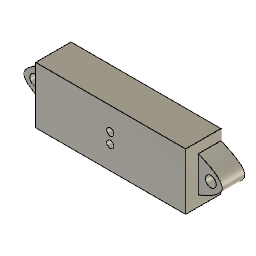
Distance Sensor (Autodesk Fusion 360 design; units mm, degrees)
Autodesk Fusion 360 part; units mm, degrees
note: some values were not read from the file. Set by a fixed rule: which sketch regions a step uses.
sketch "Sketch2" plane through (0, 0, 0) normal (0, 1, 0) x (1, 0, 0)
  line L0 (0, 0) -> (42.015, 0)
  line L1 (42.015, 0) -> (42.015, -15.89)
  line L2 (42.015, -15.89) -> (0, -15.89)
  line L3 (0, -15.89) -> (0, 0)
  circle A0 centre (45.515, -7.945) radius 1.5
  line L4 (42.015, -7.945) -> (48.69, -7.945)
  spline S0 degree 5 poles (42.015, -12.945) (42.5156, -12.7419) (43.4745, -12.3366) (44.7863, -11.7309) (46.2763, -10.9278) (47.6689, -9.93) (48.5399, -8.9364) (48.8392, -7.945) (48.5399, -6.9536) (47.6689, -5.96) (46.2763, -4.9622) (44.7863, -4.1591) (43.4745, -3.5534) (42.5156, -3.1481) (42.015, -2.945) knots 0 0 0 0 0 0 0.1 0.2 0.3 0.4 0.5 0.6 0.7 0.8 0.9 1 1 1 1 1 1
  line L5 (20.92, -15.89) -> (20.92, 0)
  spline S1 degree 5 poles (-0.175, -12.945) (-0.6756, -12.7419) (-1.6345, -12.3366) (-2.9463, -11.7309) (-4.4363, -10.9278) (-5.8289, -9.93) (-6.6999, -8.9364) (-6.9992, -7.945) (-6.6999, -6.9536) (-5.8289, -5.96) (-4.4363, -4.9622) (-2.9463, -4.1591) (-1.6345, -3.5534) (-0.6756, -3.1481) (-0.175, -2.945) knots 0 0 0 0 0 0 0.1 0.2 0.3 0.4 0.5 0.6 0.7 0.8 0.9 1 1 1 1 1 1
  line L6 (40.2192, -13.6735) -> (43.8108, -12.2165)
  line L7 (43.8108, -3.6735) -> (40.2192, -2.2165)
  line L8 (1.6208, -13.6735) -> (-1.9708, -12.2165)
  line L9 (-1.9708, -3.6735) -> (1.6208, -2.2165)
  circle A1 centre (-3.675, -7.945) radius 1.5
  line L10 (-0.175, -7.945) -> (-6.85, -7.945)
  circle A2 centre (20.92, -9.45) radius 1
  circle A3 centre (20.92, -6.45) radius 1
  line L11 (-0.175, -12.945) -> (0, -13.016)
  line L12 (-0.175, -7.945) -> (0, -7.945)
  line L13 (-0.175, -2.945) -> (0, -2.874)
  dimension "d2" = 15.89
  dimension "d3" = 3
  dimension "d5" = 3.5
  dimension "d6" = 10
  dimension "d7" = 2.945
  dimension "d8" = 15.89
  dimension "d19" = 2
  dimension "d20" = 2
  dimension "d21" = 3
  dimension "d22" = 6.45
  dimension "d25" = 49.19
  dimension "d26" = 42.19
  dimension "d27" = 55.54
  dimension "d29" = 7.945
  constraint horizontal L0
  constraint vertical L1
  constraint horizontal L2
  constraint vertical L3
  constraint coincident L0.start L3.end
  constraint midpoint L1 L4.start
  constraint perpendicular L1 L4
  constraint coincident L1 S0.start
  constraint coincident L1 S0.end
  constraint coincident L2 L5.start
  constraint coincident L0 L5.end
  constraint perpendicular L0 L5
  constraint midpoint S0.start L6
  constraint midpoint S0.end L7
  constraint symmetric A0 L5 A1
  constraint symmetric L4.start L5 L10.start
  constraint symmetric L4.end L5 L10.end
  constraint symmetric S0.start L5 S1.start
  constraint symmetric S0.end L5 S1.end
  constraint symmetric L5 L6.start L8.start
  constraint symmetric L5 L6.end L8.end
  constraint symmetric L5 L7.start L9.start
  constraint symmetric L5 L7.end L9.end
  constraint coincident L5 A2.centre
  constraint coincident L5 A3.centre
  constraint coincident L8 L11.end
  constraint coincident L3 L11.end
  constraint midpoint L3 L12.end
  constraint perpendicular L3 L12
  constraint coincident L9 L13.end
  constraint coincident L3 L13.end
  measures "d2" distance of L0.start L2.end
  measures "d3" diameter of A0
  measures "d5" distance of L1 A0.centre
  measures "d6" distance of S0.start S0.end
  measures "d7" distance of L2 S0.start
  measures "d8" distance of L0.end L1.end
  measures "d19" diameter of A2
  measures "d20" diameter of A3
  measures "d21" distance of A2.centre A3.centre
  measures "d22" distance of L0 A3.centre
  measures "d25" distance of A0.centre A1.centre
  measures "d26" distance of L4.start L10.start
  measures "d27" distance of L4.end L10.end
  measures "d29" distance of L0 A1.centre
extrude "Extrude1" add sketch "Sketch2" along normal blind 6.35 contours L0 L2 L3 L5 A2 A3 | L0 L1 L2 L5 A2 A3 | L3 S1 L9 A1 L10 L12 L13 | L5 A3 | L5 A3 | L3 S1 L8 A1 L10 L11 L12 | L1 A0 L4 S0 | L1 A0 L4 S0 | L5 A2 | L5 A2
extrude "Extrude2" add sketch "Sketch2" against normal blind 3.56 contours L0 L2 L3 L5 A2 A3 | L0 L1 L2 L5 A2 A3 | L5 A3 | L5 A3 | L5 A2 | L5 A2
extrude "Extrude3" cut sketch "Sketch2" against normal blind 25 contours L5 A3 | L5 A3 | L5 A2 | L5 A2
equation "d4 = 6.5 mm"
equation "d5 = d4 - 1.5 mm - d3 / 2"
equation "d7 = ( d8 - d6 ) / 2"
equation "d12 = -9.91 mm + 6.35 mm"
equation "d29 = d2 / 2"
